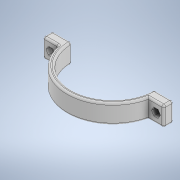
# Autodesk Inventor part: ur5e_cable_tube_bottom_85mm
Saved by Autodesk Inventor 2020 (Build 240168000, 168)
## iProperties
Created: 2021-03-04
Part Number: ur5e_cable_tube_bottom_85mm
Material: Generic
Document SubType Name: Modeling
Designer: NILY
Density: 1 g/cm^3
Appearance: Default
Author: NILY
Autodesk Inventor part; units mm, degrees
ref_plane "XZ Plane" through (0, 0, 0) normal (0, 1, 0) x (-1, 0, 0)
ref_plane "XY Plane" through (0, 0, 0) normal (0, 0, 1) x (1, 0, 0)
sketch "Sketch1" plane through (0, 0, 0) normal (0, 1, 0) x (-1, 0, 0)
  circle A0 centre (0, 0) radius 47.5
  dimension "d0" = 95
  constraints: 1 centre point, 1 coincident
  measures "d0" diameter of A0
extrude "Extrusion1" add sketch "Sketch1" along normal blind 20
shell "Shell1" thickness 5 removed faces 2 at (-10.3648, 20, 5.7529) at (-10.3648, 0, 5.7529)
sketch "Sketch2" plane through (0, 20, 0) normal (0, 1, 0) x (1, 0, 0)
  line L0 (-62.0625, 51.3519) -> (57.6609, 51.3519)
  line L1 (57.6609, 51.3519) -> (57.6609, 0)
  line L2 (57.6609, 0) -> (-62.0625, 0)
  line L3 (-62.0625, 0) -> (-62.0625, 51.3519)
  point P0 (0, 0)
  constraints: 8 end point, 2 parallel, 1 horizontal, 1 perpendicular
extrude "Extrusion2" cut sketch "Sketch2" against normal through all
ref_plane "Work Plane1" through (-47.5, 0, 0) normal (1, 0, 0) x (0, 1, 0)
sketch "Sketch3" plane through (-47.5, 0, 0) normal (1, 0, 0) x (0, 1, 0)
  line L0 (0, 0) -> (0, 47.5) projected
  line L1 (0, 0) -> (20, 0)
  line L2 (20, 0) -> (20, 10)
  line L3 (20, 10) -> (0, 10)
  line L4 (0, 10) -> (0, 0)
  point P0 (0, 10)
  dimension "d7" = 20
  dimension "d8" = 10
  constraints: 8 end point, 2 parallel, 1 horizontal, 1 perpendicular
  measures "d7" distance of L3.end L2.end
  measures "d8" distance of L2.end L1.end
extrude "Extrusion3" add sketch "Sketch3" along normal blind 2 and the other way blind 15
mirror "Mirror1" about plane through (0, 0, 0) normal (1, 0, 0) of "Extrusion3"
sketch "Sketch6" plane through (-62.5, 20, 10) normal (0, 0, 1) x (1, 0, 0)
  line L0 (10.3322, -14.0055) -> (5.7134, -13.9945)
  line L1 (5.7134, -13.9945) -> (3.4135, -9.9891)
  line L2 (3.4135, -9.9891) -> (5.7324, -5.9945)
  line L3 (5.7324, -5.9945) -> (10.3512, -6.0055)
  line L4 (10.3512, -6.0055) -> (12.6511, -10.0109)
  line L5 (12.6511, -10.0109) -> (10.3322, -14.0055)
  line L6 (0, -20) -> (0, 0) projected
  line L7 (16.0646, 0) -> (0, 0) projected
  point P0 (62.5, -20)
  point P1 (8.0323, -10)
  point P2 (0, -10)
  point P3 (8.0323, 0)
  dimension "d27" = 8
  constraints: 12 end point, 2 midpoint, 1 horizontal alignment, 1 vertical alignment, 13 other
  measures "d27" distance between parallel lines of L1 L4
extrude "Extrusion4" cut sketch "Sketch6" against normal blind 5
sketch "Sketch7" plane through (-62.5, 20, 5) normal (0, 0, 1) x (1, 0, 0)
  line L0 (0, -20) -> (0, 0) projected
  line L1 (16.0646, 0) -> (0, 0) projected
  point P0 (62.5, -20)
  point P1 (8.0323, -10)
  point P2 (0, -10)
  point P3 (8.0323, 0)
  constraints: 2 midpoint, 1 horizontal alignment, 1 vertical alignment
hole "Hole3" at (-54.4677, 10, 5) direction (0, 0, -1) diameter 5.5 end through all clearance for "Hex Head Bolt" size "M5" standard "Ansi Metric M Profile"
mirror "Mirror3" about plane through (0, 0, 0) normal (1, 0, 0) of "Extrusion4", "Hole3"
fillet "Fillet1" radius 2 23 edges at (-62.5, 0, 5) (-62.5, 20, 5) (-46.4354, 10, 10) (-54.4677, 0, 10) (-62.5, 10, 10) (-54.4677, 20, 10) (0, 20, 47.5) (0, 20, 42.5) (0, 0, 47.5) (-52.5, 20, 0) (52.5, 20, 0) (-62.5, 10, 0) (-52.5, 0, 0) (52.5, 0, 0) (0, 0, 42.5) (54.4677, 20, 10) (62.5, 10, 10) (54.4677, 0, 10) (62.5, 0, 5) (62.5, 20, 5) (62.5, 10, 0) (-42.5, 10, 0) (42.5, 10, 0)
body "Solid1"
